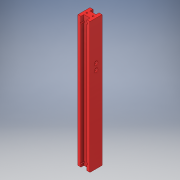
# Autodesk Inventor part: ShortBeamSplit
Saved by Autodesk Inventor 2019 (Build 230136000, 136)
## iProperties
Created: 2019-09-28
Part Number: ShortBeamSplit
Material: Generic
Document SubType Name: Modeling
Designer: james
Density: 1 g/cm^3
Appearance: Light Red
Author: james
Autodesk Inventor part; units mm, degrees
ref_plane "YZ Plane" through (0, 0, 0) normal (1, 0, 0) x (0, 1, 0)
ref_plane "XZ Plane" through (0, 0, 0) normal (0, 1, 0) x (-1, 0, 0)
ref_plane "XY Plane" through (0, 0, 0) normal (0, 0, 1) x (1, 0, 0)
sketch "Sketch1" plane through (0, 0, 0) normal (0, 1, 0) x (-1, 0, 0)
  line L0 (16.1925, 35.7868) -> (-9.2075, 35.7868)
  line L1 (-9.2075, 35.7868) -> (-9.2075, 10.3868)
  line L2 (-9.2075, 10.3868) -> (16.1925, 10.3868)
  line L3 (16.1925, 10.3868) -> (16.1925, 35.7868)
  point P0 (0, 0)
  dimension "d0" = 25.4
  dimension "d1" = 25.4
  constraints: 8 end point, 2 parallel, 1 horizontal, 1 perpendicular
  measures "d0" distance of L0.start L0.end
  measures "d1" distance of L0.end L1.end
extrude "Extrusion1" add sketch "Sketch1" along normal blind 274.955
sketch "Sketch2" plane through (0, 274.955, 0) normal (0, 1, 0) x (1, 0, 0)
  line L0 (-9.8425, -16.7368) -> (2.8575, -16.7368)
  line L1 (2.8575, -16.7368) -> (2.8575, -1.003)
  line L2 (2.8575, -1.003) -> (-9.8425, -1.003)
  line L3 (-9.8425, -1.003) -> (-9.8425, -16.7368)
  line L4 (9.2075, -35.7868) -> (9.2075, -10.3868) projected
  line L5 (-16.1925, -10.3868) -> (-16.1925, -35.7868) projected
  line L6 (9.2075, -10.3868) -> (-16.1925, -10.3868) projected
  point P0 (0, 0)
  dimension "d4" = 6.35
  dimension "d5" = 6.35
  dimension "d6" = 6.35
  constraints: 8 end point, 2 parallel, 1 horizontal, 1 perpendicular
  measures "d4" distance between parallel lines of L1 L4
  measures "d5" distance between parallel lines of L5 L3
  measures "d6" distance between parallel lines of L0 L6
extrude "Extrusion2" cut sketch "Sketch2" against normal blind 508
sketch "Sketch4" plane through (0, 274.955, 0) normal (0, 1, 0) x (1, 0, 0)
  line L0 (-9.8425, -29.4368) -> (2.8575, -29.4368)
  line L1 (2.8575, -29.4368) -> (2.8575, -45.8861)
  line L2 (2.8575, -45.8861) -> (-9.8425, -45.8861)
  line L3 (-9.8425, -45.8861) -> (-9.8425, -29.4368)
  line L4 (-16.1925, -10.3868) -> (-16.1925, -35.7868) projected
  line L5 (9.2075, -35.7868) -> (9.2075, -10.3868) projected
  line L6 (-16.1925, -35.7868) -> (9.2075, -35.7868) projected
  point P0 (0, 0)
  dimension "d20" = 6.35
  dimension "d21" = 6.35
  dimension "d22" = 6.35
  constraints: 8 end point, 2 parallel, 1 horizontal, 1 perpendicular
  measures "d20" distance between parallel lines of L3 L4
  measures "d21" distance between parallel lines of L5 L1
  measures "d22" distance between parallel lines of L6 L0
extrude "Extrusion3" cut sketch "Sketch4" against normal blind 508
sketch "Sketch5" plane through (9.2075, 0, 10.3868) normal (0, 0, -1) x (-1, 0, 0)
  line L0 (0, 0) -> (6.35, 0) projected
  line L1 (0, 0) -> (0, 274.955) projected
  line L2 (25.4, 0) -> (25.4, 274.955) projected
  line L3 (19.05, 0) -> (25.4, 0) projected
  point P0 (9.2075, 0)
  point P1 (19.05, 6.35)
  point P2 (6.35, 12.7)
  dimension "d25" = 12.7
  dimension "d27" = 6.35
  dimension "d28" = 6.35
  dimension "d60" = 19.05
  measures "d25" distance from line of L0 point (6.35, 12.7)
  measures "d27" distance from line of L2 point (19.05, 6.35)
  measures "d28" distance from line of L3 point (19.05, 6.35)
  measures "d60" distance from line of point (6.35, 12.7) L2
hole "Hole2" at (-9.8425, 6.35, 10.3868) at (2.8575, 12.7, 10.3868) direction (0, 0, 1) diameter 3.175 end through all
sketch "Sketch6" plane through (-16.1925, 0, 10.3868) normal (0, 0, -1) x (-1, 0, 0)
  line L0 (-6.35, 274.955) -> (-6.35, 7.9375) projected
  line L1 (-25.4, 274.955) -> (-19.05, 274.955) projected
  line L2 (-25.4, 0) -> (-25.4, 274.955) projected
  line L3 (-6.35, 274.955) -> (0, 274.955) projected
  line L4 (0, 0) -> (0, 274.955) projected
  point P0 (-16.1925, 0)
  point P1 (-19.05, 268.605)
  point P2 (-6.35, 262.255)
  dimension "d36" = 6.35
  dimension "d38" = 12.7
  dimension "d58" = 6.35
  dimension "d59" = 19.05
  constraints: 1 point on line
  measures "d36" distance from line of point (-19.05, 268.605) L1
  measures "d38" distance from line of L3 point (-6.35, 262.255)
  measures "d58" distance from line of L4 point (-6.35, 262.255)
  measures "d59" distance from line of point (-19.05, 268.605) L4
hole "Hole3" at (2.8575, 268.605, 10.3868) at (-9.8425, 262.255, 10.3868) direction (0, 0, 1) diameter 3.175 end through all
sketch "Sketch7" plane through (0, 0, 0) normal (0, -1, 0) x (1, 0, 0)
  line L0 (2.8575, 35.7868) -> (9.2075, 35.7868) projected
  line L1 (9.2075, 35.7868) -> (9.2075, 10.3868) projected
  line L2 (-16.1925, 10.3868) -> (-16.1925, 35.7868) projected
  line L3 (-16.1925, 35.7868) -> (-9.8425, 35.7868) projected
  point P0 (0, 0)
  point P1 (-9.8425, 23.0868)
  point P2 (2.8575, 23.0868)
  dimension "d47" = 12.7
  dimension "d48" = 6.35
  dimension "d49" = 6.35
  dimension "d50" = 12.7
  measures "d47" distance from line of L0 point (2.857, 23.087)
  measures "d48" distance from line of L1 point (2.857, 23.087)
  measures "d49" distance from line of L2 point (-9.843, 23.087)
  measures "d50" distance from line of L3 point (-9.843, 23.087)
hole "Hole4" at (-9.8425, 0, 23.0868) at (2.8575, 0, 23.0868) direction (0, 1, 0) diameter 3.175 end through all
sketch "Sketch13" plane through (9.2075, 274.955, 35.7868) normal (1, 0, 0) x (0, 0, -1)
  line L0 (0, 0) -> (25.4, 0) projected
  line L1 (0, -274.955) -> (0, 0) projected
  point P0 (35.7868, -274.955)
  point P1 (12.7, -82.55)
  point P2 (12.7, -95.25)
  point P3 (0, -88.8492)
  dimension "d95" = 82.55
  dimension "d96" = 12.7
  dimension "d97" = 12.7
  dimension "d98" = 12.7
  measures "d95" distance from line of point (12.7, -82.55) L0
  measures "d96" distance from line of L1 point (12.7, -82.55)
  measures "d97" distance from line of L1 point (12.7, -95.25)
  measures "d98" distance of point (12.7, -95.25) point (12.7, -82.55)
hole "Hole6" at (9.2075, 192.405, 23.0868) at (9.2075, 179.705, 23.0868) direction (-1, 0, 0) diameter 4.4958 end through all countersink diameter 8.4328 countersink angle 82 clearance for "Flat Head Machine Screw (82)" size "#8" standard "Ansi Unified Screw Threads"
body "Solid1"
